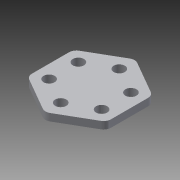
# Autodesk Inventor part: Roller Pneumatic Back Connector (Custom)
Saved by Autodesk Inventor 2014 (Build 180170000, 170)
## iProperties
Created: 2014-01-06
Part Number: Roller Pneumatic Back Connector (Custom)
Material: Aluminum 6061
Document SubType Name: Modeling
Designer: Andrew Toennies
Density: 7.85 g/cm^3
Appearance: Aluminum - Flat
Mass: 11.2814 g
Surface Area: 21.4027 cm^2
Volume: 1.43712 cm^3
Author: Andrew Toennies
Autodesk Inventor part; units mm, degrees
ref_plane "YZ Plane" through (0, 0, 0) normal (1, 0, 0) x (0, 1, 0)
ref_plane "XZ Plane" through (0, 0, 0) normal (0, 1, 0) x (-1, 0, 0)
ref_plane "XY Plane" through (0, 0, 0) normal (0, 0, 1) x (1, 0, 0)
sketch "Sketch1" plane through (0, 0, 0) normal (0, 1, 0) x (-1, 0, 0)
  circle A0 centre (0, 0) radius 2.413
  circle A1 centre (0, 25.4) radius 2.413
  line L0 (0, 25.4) -> (0, 0) construction
  circle A2 centre (11.3919, 19.05) radius 2.413
  circle A3 centre (11.3919, 6.35) radius 2.413
  circle A4 centre (-11.3919, 6.35) radius 2.413
  circle A5 centre (-11.3919, 19.05) radius 2.413
  line L1 (-11.3919, 6.35) -> (-11.3919, 19.05) construction
  line L2 (-11.3919, 19.05) -> (11.3919, 19.05) construction
  line L3 (1.5875, 31.5808) -> (15.5575, 23.5152)
  line L4 (17.145, 20.7656) -> (17.145, 4.6344)
  line L5 (15.5575, 1.8848) -> (1.5875, -6.1808)
  line L6 (-1.5875, -6.1808) -> (-15.5575, 1.8848)
  line L7 (-17.145, 4.6344) -> (-17.145, 20.7656)
  line L8 (-15.5575, 23.5152) -> (-1.5875, 31.5808)
  arc A6 (1.5875, 31.5808) -> (-1.5875, 31.5808) centre (0, 28.8312) ccw
  arc A7 (-15.5575, 23.5152) -> (-17.145, 20.7656) centre (-13.97, 20.7656) ccw
  arc A8 (-17.145, 4.6344) -> (-15.5575, 1.8848) centre (-13.97, 4.6344) ccw
  arc A9 (-1.5875, -6.1808) -> (1.5875, -6.1808) centre (0, -3.4312) ccw
  arc A10 (15.5575, 1.8848) -> (17.145, 4.6344) centre (13.97, 4.6344) ccw
  arc A11 (17.145, 20.7656) -> (15.5575, 23.5152) centre (13.97, 20.7656) ccw
  point P0 (0, 12.7)
  point P1 (0, 32.4973)
  point P2 (17.145, 22.5987)
  point P3 (17.145, 2.8013)
  point P4 (0, -7.0973)
  point P5 (-17.145, 2.8013)
  point P6 (-17.145, 22.5987)
  dimension "d1" = 4.826
  dimension "d2" = 25.4
  dimension "d3" = 4.826
  dimension "d4" = 4.826
  dimension "d5" = 12.7
  dimension "d6" = 11.3919
  dimension "d7" = 11.3919
  dimension "d8" = 6.35
  dimension "d9" = 4.826
  dimension "d10" = 4.826
  dimension "d11" = 11.3919
  dimension "d12" = 12.7
  dimension "d13" = 34.29
  dimension "d14" = 3.175
  constraints: 18 end point, 13 point on line, 12 centre point, 12 point on circle, 12 tangent, 6 equal radius, 1 coincident, 1 midpoint, 1 parallel, 1 perpendicular, 1 vertical, 13 other
  measures "d1" diameter of A1
  measures "d2" distance of L0.start L0.end
  measures "d3" diameter of A2
  measures "d4" diameter of A3
  measures "d5" distance of A3.centre L2.end
  measures "d6" distance from line of L0 A3.centre
  measures "d7" distance from line of L0 L2.end
  measures "d8" vertical distance of point (0, 0) A3.centre
  measures "d9" diameter of A4
  measures "d10" diameter of A5
  measures "d11" distance between parallel lines of L1 L0
  measures "d12" distance of L1.start L1.end
  measures "d13" distance between parallel lines of L7 L4
  measures "d14" radius of A6
extrude "Extrusion1" add sketch "Sketch1" along normal blind 3.175
equation "\"d7\" = d6"
equation "\"d11\" = d6"
body "Solid1"
